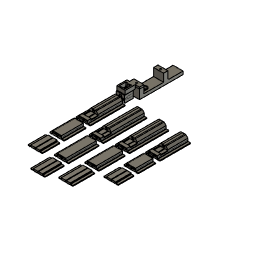
FlexiaGlove (Autodesk Fusion 360 design; units mm, degrees)
Autodesk Fusion 360 part; units mm, degrees
note: some values were not read from the file. Chosen so that the rebuilt part matches the saved one: which face or edge a step refers to. Set by a fixed rule: which sketch regions a step uses.
(part 1 of 2)
sketch "Sketch1" plane through (0, 0, 0) normal (0, 0, 1) x (1, 0, 0) in component "Flex Sensor Mount"
  line L0 (-4.7625, -1.75) -> (4.7625, -1.75)
  line L1 (4.7625, -1.75) -> (4.7625, 6.2)
  line L2 (-4.7625, 6.2) -> (-4.7625, -1.75)
  line L3 (-0.3, 0.4) -> (0.3, 0.4)
  line L4 (0.3, 0.4) -> (0.3, -0.4)
  line L5 (0.3, -0.4) -> (-0.3, -0.4)
  line L6 (-0.3, -0.4) -> (-0.3, 0.4)
  line L7 (-4.0625, 3.25) -> (4.0625, 3.25)
  line L8 (4.0625, 3.25) -> (4.0625, 0.75)
  line L9 (4.0625, 0.75) -> (-4.0625, 0.75)
  line L10 (-4.0625, 0.75) -> (-4.0625, 3.25)
  line L11 (-4.7625, 6.2) -> (4.7625, 6.2)
  dimension "d283" = 0.8
  dimension "d284" = 0.6
  dimension "d285" = 0.3
  dimension "d286" = 0.4
  dimension "d287" = 2.5
  dimension "d289" = 4.7625
  dimension "d291" = 1.75
  dimension "d293" = 0.35
  dimension "d294" = 8.125
  dimension "d296" = 9.525
  dimension "d297" = 4.0625
  dimension "d368" = 7.95
  constraint horizontal L0
  constraint vertical L1
  constraint vertical L2
  constraint horizontal L3
  constraint vertical L4
  constraint horizontal L5
  constraint vertical L6
  constraint horizontal L7
  constraint vertical L8
  constraint horizontal L9
  constraint vertical L10
  constraint horizontal L11
  measures "d283" distance of L3.start L5.end
  measures "d284" distance of L4.end L5.end
  measures "d285" distance of origin L6
  measures "d286" distance of origin L3
  measures "d287" distance of L7.end L8.end
  measures "d289" distance of origin L2
  measures "d291" distance of origin L0
  measures "d293" distance of L3 L9
  measures "d294" distance of L7.start L7.end
  measures "d296" distance of L0.start L0.end
  measures "d297" distance of origin L10
  measures "d368" distance of L0 L11
extrude "Extrude1" add sketch "Sketch1" along normal blind 12 from surface at 40.25 makes body 1 in component "Flex Sensor Mount"
sketch "Sketch3" plane through (0, 0, 52.25) normal (0, 0, 1) x (1, 0, 0) in component "Flex Sensor Mount"
  line L0 (0.3, -0.4) -> (-0.3, -0.4)
  line L1 (-0.3, -0.4) -> (-0.3, 0.4)
  line L2 (-0.3, 0.4) -> (0.3, 0.4)
  line L3 (0.3, 0.4) -> (0.3, -0.4)
  line L4 (4.0625, 0.75) -> (-4.0625, 0.75)
  line L5 (-4.0625, 0.75) -> (-4.0625, 3.25)
  line L6 (-4.0625, 3.25) -> (4.0625, 3.25)
  line L7 (4.0625, 3.25) -> (4.0625, 0.75)
  line L8 (-4.7625, 6.2) -> (-4.7625, -1.75)
  line L9 (-4.7625, -1.75) -> (4.7625, -1.75)
  line L10 (4.7625, -1.75) -> (4.7625, 6.2)
  line L11 (-4.0625, 2.5) -> (4.0625, 2.5)
  line L12 (4.0625, 2.5) -> (4.0625, 1.25)
  line L13 (4.0625, 1.25) -> (-4.0625, 1.25)
  line L14 (-4.0625, 1.25) -> (-4.0625, 2.5)
  line L15 (4.7625, 6.2) -> (-4.7625, 6.2)
  dimension "d305" = 1.25
  dimension "d312" = 0.75
  constraint horizontal L11
  constraint vertical L12
  constraint horizontal L13
  constraint vertical L14
  constraint coincident L7 L12.end
  constraint coincident L5 L11.start
  measures "d305" distance of L11.start L13.end
  measures "d312" distance of L6 L11
extrude "Extrude3" add sketch "Sketch3" against normal blind 4 contours L4 L5 L7 L13 | L5 L6 L7 L11 bodies 1 in component "Flex Sensor Mount"
sketch "Sketch2" plane through (0, 6.2, 0) normal (0, 1, 0) x (-1, 0, 0) in component "Flex Sensor Mount"
  line L0 (-4.7625, 40.25) -> (4.7625, 40.25)
  line L1 (4.7625, 40.25) -> (4.7625, 52.25)
  line L2 (4.7625, 52.25) -> (-4.7625, 52.25)
  line L3 (-4.7625, 52.25) -> (-4.7625, 40.25)
  line L4 (-4.0625, 40.25) -> (4.0625, 40.25)
  line L5 (4.0625, 40.25) -> (4.0625, 48.25)
  line L6 (-4.0625, 48.25) -> (-4.0625, 40.25)
  line L7 (4.0625, 52.25) -> (-4.0625, 52.25)
  line L8 (4.7625, 42.25) -> (-4.7625, 42.25)
  circle A0 centre (0, 46.9204) radius 6.6704
  line L9 (4.0625, 48.25) -> (-4.0625, 48.25)
  line L10 (-4.7625, 40.25) -> (4.7625, 40.25)
  line L11 (4.7625, 40.25) -> (4.7625, 52.25)
  line L12 (4.7625, 52.25) -> (-4.7625, 52.25)
  line L13 (-4.7625, 52.25) -> (-4.7625, 40.25)
  dimension "d302" = 2
  constraint coincident L5 L7.start
  constraint coincident L6 L7.end
  constraint perpendicular L6 L7
  constraint coincident L1 L8.start
  constraint coincident L3 L8.end
  constraint perpendicular L3 L8
  constraint coincident L8.start A0
  constraint tangent L0 A0
  constraint coincident L8.end A0
  measures "d302" distance of L0 L8
extrude "Extrude2" cut sketch "Sketch2" against normal up to surface (7.95 mm away) contours L0 L3 L6 A0 L10 L13 | L0 L4 L6 A0 L10 | L0 L4 L5 A0 L10 | L0 L1 L5 A0 L10 L11 bodies 1 in component "Flex Sensor Mount"
sketch "Sketch4" plane through (0, 6.2, 0) normal (0, 1, 0) x (-1, 0, 0) in component "Flex Sensor Mount"
  arc A0 (-4.7625, 42.25) -> (4.7625, 42.25) centre (0, 46.9204) ccw
  line L0 (4.7625, 42.25) -> (4.7625, 52.25)
  line L1 (4.7625, 52.25) -> (-4.7625, 52.25)
  line L2 (-4.7625, 52.25) -> (-4.7625, 42.25)
  circle A1 centre (0, 46.9204) radius 3.25
  line L3 (2.3452, 44.6704) -> (-2.3452, 44.6704)
  arc A2 (-4.7625, 42.25) -> (4.7625, 42.25) centre (0, 46.9204) ccw
  line L4 (4.7625, 42.25) -> (4.7625, 52.25)
  line L5 (4.7625, 52.25) -> (-4.7625, 52.25)
  line L6 (-4.7625, 52.25) -> (-4.7625, 42.25)
  dimension "d313" = 6.5
  dimension "d314" = 2.25
  constraint concentric A0 A1
  constraint coincident A1 L3.start
  constraint coincident A1 L3.end
  constraint horizontal L3
  measures "d313" diameter of A1
  measures "d314" distance of A0.centre L3
extrude "Extrude4" cut sketch "Sketch4" against normal blind 2.5 contours A1 L3 picked at (0.4352, 46.4124) bodies 1 in component "Flex Sensor Mount"
chamfer "Chamfer1" distance 0.1 angle 45 2 edges at (0, 6.2, 50.1704) (0, 6.2, 44.6704) on bodies 1 in component "Flex Sensor Mount"
sketch "Sketch1 (2)" plane through (0, 0, 0) normal (0, 0, 1) x (1, 0, 0) in component "Base"
  line L0 (-1.75, 1.75) -> (9.75, 1.75)
  line L1 (9.75, 1.75) -> (9.75, -1.75)
  line L2 (9.75, -1.75) -> (-1.75, -1.75)
  line L3 (-1.75, -1.75) -> (-1.75, 1.75)
  line L4 (-1.75, 1) -> (-0.25, 1)
  line L5 (-0.25, 1) -> (-0.25, -0.75)
  line L6 (-0.25, -0.75) -> (-1.75, -0.75)
  line L7 (-1.75, -0.75) -> (-1.75, 1)
  line L8 (9.75, 1) -> (8.25, 1)
  line L9 (8.25, 1) -> (8.25, -0.75)
  line L10 (8.25, -0.75) -> (9.75, -0.75)
  line L11 (9.75, -0.75) -> (9.75, 1)
  line L12 (-0.3, 0.4) -> (0.3, 0.4)
  line L13 (0.3, 0.4) -> (0.3, -0.4)
  line L14 (0.3, -0.4) -> (-0.3, -0.4)
  line L15 (-0.3, -0.4) -> (-0.3, 0.4)
  dimension "d1" = 11.5
  dimension "d4" = 1.75
  dimension "d77" = 1.75
  dimension "d79" = 1.5
  dimension "d80" = 1.75
  dimension "d81" = 1.5
  dimension "d83" = 1
  dimension "d84" = 1
  dimension "d86" = 3.5
  dimension "d87" = 1.75
  dimension "d131" = 0.6
  dimension "d132" = 0.8
  dimension "d133" = 0.3
  dimension "d134" = 0.4
  constraint horizontal L0
  constraint vertical L1
  constraint horizontal L2
  constraint vertical L3
  constraint horizontal L4
  constraint vertical L5
  constraint horizontal L6
  constraint vertical L7
  constraint coincident L3 L4.start
  constraint horizontal L8
  constraint vertical L9
  constraint horizontal L10
  constraint vertical L11
  constraint coincident L1 L8.start
  constraint horizontal L12
  constraint vertical L13
  constraint horizontal L14
  constraint vertical L15
  measures "d1" distance of L1.end L2.end
  measures "d4" distance of origin L3
  measures "d77" distance of L4.end L5.end
  measures "d79" distance of L4.start L4.end
  measures "d80" distance of L8.end L9.end
  measures "d81" distance of L8.start L8.end
  measures "d83" distance of L2 L10
  measures "d84" distance of L2 L6
  measures "d86" distance of L0 L2
  measures "d87" distance of origin L2
  measures "d131" distance of L12.start L12.end
  measures "d132" distance of L12.end L13.end
  measures "d133" distance of origin L15
  measures "d134" distance of origin L14
extrude "Extrude1'" add sketch "Sketch1 (2)" along normal blind 40 separate body contours L0 L1 L2 L3 L4 L5 L6 L8 L9 L10 L12 L13 L14 | L3 L4 L5 L6 L7 L12 L14 L15 | L1 L8 L9 L10 L11 makes body 2 in component "Base"
sketch "Sketch2 (2)" plane through (0, 1.75, 0) normal (0, 1, 0) x (-1, 0, 0) in component "Base"
  line L0 (-9.75, 0) -> (1.75, 0)
  line L1 (1.75, 0) -> (1.75, 40)
  line L2 (1.75, 40) -> (-9.75, 40)
  line L3 (-9.75, 40) -> (-9.75, 0)
  line L4 (-9.75, 40) -> (1.75, 40)
  line L5 (1.75, 40) -> (1.75, 35)
  line L6 (1.75, 35) -> (-9.75, 35)
  line L7 (-9.75, 35) -> (-9.75, 40)
  line L8 (-9.75, 12.4) -> (1.75, 12.4)
  line L9 (1.75, 12.4) -> (1.75, 7.4)
  line L10 (1.75, 7.4) -> (-9.75, 7.4)
  line L11 (-9.75, 7.4) -> (-9.75, 12.4)
  circle A0 centre (-4, 37.6385) radius 0.95
  circle A1 centre (-4, 10.0385) radius 0.95
  line L12 (-1.0736, 23.3752) -> (-1.0736, 24.3004)
  line L13 (-6.8236, 23.3752) -> (-6.8236, 24.241)
  arc A2 (-6.8236, 23.3752) -> (-1.0736, 23.3752) centre (-3.9486, 23.3752) ccw
  arc A3 (-1.0736, 24.3004) -> (-6.8236, 24.241) centre (-4, 29.25) ccw
  line L14 (-3.9486, 20.5002) -> (-4, 12.4)
  dimension "d8" = 11.5
  dimension "d9" = 11.5
  dimension "d10" = 5
  dimension "d11" = 5
  dimension "d12" = 27.6
  dimension "d13" = 22.6
  dimension "d15" = 5.75
  dimension "d16" = 5.75
  dimension "d17" = 1.9
  dimension "d18" = 1.9
  dimension "d47" = 5.75
  dimension "d48" = 11.5
  dimension "d49" = 5.75
  dimension "d50" = 5.875
  constraint horizontal L4
  constraint vertical L5
  constraint horizontal L6
  constraint vertical L7
  constraint coincident L2.end L3.start
  constraint horizontal L8
  constraint vertical L9
  constraint horizontal L10
  constraint vertical L11
  constraint coincident L3 L8.start
  constraint tangent L6 A3
  constraint vertical L12
  constraint vertical L13
  constraint tangent L12 A2
  constraint tangent L13 A2
  constraint midpoint A2 L14.start
  constraint midpoint L8 L14.end
  measures "d8" distance of L5.end L6.end
  measures "d9" distance of L9.end L10.end
  measures "d10" distance of L8.start L10.end
  measures "d11" distance of L2.end L6.end
  measures "d12" distance of A0.centre A1.centre
  measures "d13" distance of L6 L8
  measures "d15" horizontal distance of L2.end A0.centre
  measures "d16" distance of L11 A1.centre
  measures "d17" diameter of A0
  measures "d18" diameter of A1
  measures "d47" distance of L3 A3.centre
  measures "d48" diameter of A3
  measures "d49" diameter of A2
  measures "d50" distance of A3.centre A2.centre
extrude "Extrude1''" add sketch "Sketch2 (2)" along normal blind 9 contours L1 L3 L8 L9 L10 L11 | L1 L2 L3 L4 L5 L6 L7 bodies 2 in component "Base"
sketch "Sketch4 (2)" plane through (0, 1.75, 0) normal (0, 1, 0) x (-1, 0, 0) in component "Base"
  line L0 (1.75, 12.4) -> (1.75, 35)
  line L1 (1.75, 35) -> (-9.75, 35)
  line L2 (-9.75, 35) -> (-9.75, 12.4)
  line L3 (0.3, 24.6) -> (-9.75, 24.6)
  line L4 (0.3, 34.9) -> (-9.75, 34.9)
  line L5 (0.3, 34.9) -> (0.3, 24.6)
  line L6 (-9.75, 28.9) -> (-4, 28.9)
  circle A0 centre (-4, 28.9) radius 2.375
  circle A1 centre (-4, 28.9) radius 2.875
  line L7 (-8.3, 24.6) -> (-8.3, 34.9)
  line L8 (-9.75, 12.4) -> (1.75, 12.4)
  circle A2 centre (-4, 28.9) radius 4.3
  line L9 (-0.75, 24.6) -> (-0.75, 34.9)
  circle A3 centre (-4, 28.9) radius 3.25
  line L10 (-0.9996, 30.149) -> (0.3, 32.4)
  line L11 (-7.25, 28.9) -> (-7.25, 34.9)
  line L12 (-0.9996, 30.149) -> (-4, 28.9)
  dimension "d119" = 0.3
  dimension "d121" = 5.75
  dimension "d122" = 4.75
  dimension "d124" = 4.3
  dimension "d125" = 5.75
  dimension "d126" = 6
  dimension "d130" = 8.6
  dimension "d135" = 16.5
  dimension "d203" = 0.75
  dimension "d216" = 6.5
  dimension "d217" = 2.5
  dimension "d230" = 150
  dimension "d237" = 142.601
  constraint horizontal L4
  constraint horizontal L3
  constraint coincident L2 L3.end
  constraint coincident L2 L4.end
  constraint vertical L5
  constraint coincident L2 L6.start
  constraint perpendicular L2 L6
  constraint coincident L6.end A0.centre
  constraint coincident L3 L7.start
  constraint coincident L4 L7.end
  constraint perpendicular L4 L7
  constraint concentric A1 A2
  constraint tangent L5 A2
  constraint coincident L3 L9.start
  constraint coincident L4 L9.end
  constraint perpendicular L4 L9
  constraint concentric A2 A3
  constraint coincident A3 L10.start
  constraint coincident L5 L10.end
  constraint coincident A3 L11.start
  constraint coincident L6 L11.start
  constraint coincident L4 L11.end
  constraint tangent A3 L11
  measures "d119" distance of origin L5
  measures "d121" distance of L6.start L6.end
  measures "d122" diameter of A0
  measures "d124" distance of L3 L6
  measures "d125" diameter of A1
  measures "d126" distance of L4 L6.end
  measures "d130" distance of L5 L7
  measures "d135" distance of L6.end L8
  measures "d203" distance of origin L9
  measures "d216" diameter of A3
  measures "d217" distance of L4 L10.end
  measures "d230" angle of L5 L10
  measures "d237" angle of L10 L12
extrude "Extrude3'" cut sketch "Sketch4 (2)" against normal blind 2.85 contours L4 A2 L9 L11 | L6 A1 A3 L12 | A2 L9 A3 L10 L11 | L6 A1 A3 L12 | L4 L5 A2 L9 L10 | L6 A0 A1 L12 | L6 A0 A1 L12 | A2 L9 L10 | L6 A0 L12 | L6 A0 L12 picked at (-0.5421, 31.0649) bodies 2 in component "Base"
extrude "Extrude14" cut 1 faces at (8.15, 10.75, 37.5462) along direction (0, -1, 0) blind 2 on bodies 2 bodies 2 in component "Base"
chamfer "Chamfer1'" distance 1 angle 45 1 edges at (4, 1.75, 7.4) on bodies 2 in component "Base"
sketch "Sketch1 (3)" plane through (0, 8.75, 0) normal (0, 1, 0) x (-1, 0, 0) in component "Splay Sensor Mount"
  circle A0 centre (-4, 37.6385) radius 0.95
  line L0 (-9.75, 35) -> (1.75, 35)
  line L1 (1.75, 35) -> (1.75, 40)
  line L2 (1.75, 40) -> (-9.75, 40)
  line L3 (-9.75, 40) -> (-9.75, 35)
extrude "Extrude1'''" add sketch "Sketch1 (3)" along normal blind 2 separate body makes body 3 in component "Splay Sensor Mount"
sketch "Sketch2 (3)" plane through (0, 0, 40) normal (0, 0, 1) x (1, 0, 0) in component "Splay Sensor Mount"
  line L0 (-1.75, 8.75) -> (9.75, 8.75)
  line L1 (9.75, 8.75) -> (9.75, 10.75)
  line L2 (9.75, 10.75) -> (-1.75, 10.75)
  line L3 (-1.75, 10.75) -> (-1.75, 8.75)
  line L4 (4.7625, 10.75) -> (-4.7625, 10.75)
  line L5 (-4.7625, 10.75) -> (-4.7625, 6.25)
  line L6 (-4.7625, 6.25) -> (4.7625, 6.25)
  line L7 (4.7625, 6.25) -> (4.7625, 10.75)
  dimension "d327" = 9.525
  dimension "d328" = 4.5
  dimension "d329" = 4.7625
  constraint horizontal L4
  constraint vertical L5
  constraint horizontal L6
  constraint vertical L7
  constraint coincident L2 L4.start
  measures "d327" distance of L4.start L4.end
  measures "d328" distance of L4.start L6.end
  measures "d329" distance of origin L5
extrude "Extrude2'" add sketch "Sketch2 (3)" along normal blind 11.5 contours L0 L2 L3 L4 L7 | L0 L3 L4 L5 L6 L7 bodies 3 in component "Splay Sensor Mount"
sketch "Sketch3 (2)" plane through (0, 10.75, 0) normal (0, 1, 0) x (-1, 0, 0) in component "Splay Sensor Mount"
  circle A0 centre (-4, 37.6385) radius 0.95
  line L0 (-9.75, 40) -> (-9.75, 35)
  line L1 (-9.75, 35) -> (1.75, 35)
  line L2 (1.75, 35) -> (1.75, 40)
  line L3 (1.75, 40) -> (4.7625, 40)
  line L4 (4.7625, 40) -> (4.7625, 51.5)
  line L5 (4.7625, 51.5) -> (-4.7625, 51.5)
  line L6 (-4.7625, 51.5) -> (-4.7625, 40)
  line L7 (-4.7625, 40) -> (-9.75, 40)
  line L8 (3.25, 42.6704) -> (-3.25, 42.6704)
  line L9 (-3.25, 42.6704) -> (-3.25, 50.1704)
  line L10 (-3.25, 50.1704) -> (3.25, 50.1704)
  line L11 (3.25, 50.1704) -> (3.25, 42.6704)
  line L12 (3.25, 42.6704) -> (1, 42.6704)
  line L13 (1, 42.6704) -> (1, 43.4204)
  line L14 (1, 43.4204) -> (3.25, 43.4204)
  line L15 (3.25, 43.4204) -> (3.25, 42.6704)
  line L16 (-3.25, 42.6704) -> (-1, 42.6704)
  line L17 (-1, 42.6704) -> (-1, 43.4204)
  line L18 (-1, 43.4204) -> (-3.25, 43.4204)
  line L19 (-3.25, 43.4204) -> (-3.25, 42.6704)
  line L20 (1, 43.4204) -> (-1, 43.4204)
  arc A1 (2.3452, 44.6704) -> (-2.3452, 44.6704) centre (0, 46.9204) ccw
  dimension "d332" = 6.5
  dimension "d333" = 7.5
  dimension "d340" = 0.75
  dimension "d341" = 0.75
  dimension "d342" = 2
  dimension "d343" = 2.25
  dimension "d369" = 3.25
  dimension "d370" = 3.25
  constraint horizontal L8
  constraint vertical L9
  constraint horizontal L10
  constraint vertical L11
  constraint horizontal L12
  constraint vertical L13
  constraint horizontal L14
  constraint vertical L15
  constraint horizontal L16
  constraint vertical L17
  constraint horizontal L18
  constraint vertical L19
  measures "d332" distance of L9.end L10.end
  measures "d333" distance of L8.end L9.end
  measures "d340" distance of L16.end L17.end
  measures "d341" distance of L12.end L13.end
  measures "d342" distance of L13 L17
  measures "d343" distance of L13.end L14.end
  measures "d369" distance of L10 A1.centre
  measures "d370" distance of L11 A1.centre
extrude "Extrude3''" cut sketch "Sketch3 (2)" against normal up to surface (4.5 mm away) contours L8 L11 L12 L13 L14 L15 | L9 L11 L14 L18 L20 A1 | L8 L9 L16 L17 L18 L19 | L10 L11 A1 | L9 L10 A1 bodies 3 in component "Splay Sensor Mount"
sketch "Sketch1 (4)" plane through (0, 0, 0) normal (0, 1, 0) x (1, 0, 0) in component "Cam"
  circle A0 centre (4, -28.9) radius 2.375
  circle A1 centre (4, -28.9) radius 3.125
  line L0 (6.0041, -25.9523) -> (6.7835, -27.4795)
  line L1 (1.9959, -25.9523) -> (1.2165, -27.4795)
  line L2 (4, -28.9) -> (4, -26.975)
  line L3 (4, -28.9) -> (4, -32.525)
  line L4 (6.1835, -33.0681) -> (7.0326, -29.6543)
  line L5 (1.8165, -33.0681) -> (0.9674, -29.6543)
  arc A2 (6.0041, -25.9523) -> (1.9959, -25.9523) centre (4, -26.975) ccw
  arc A3 (1.8165, -33.0681) -> (6.1835, -33.0681) centre (4, -32.525) ccw
  arc A4 (7.25, -28.9) -> (0.9996, -30.149) centre (4, -28.9) ccw
  line L6 (0.9996, -30.149) -> (4, -28.9)
  line L7 (4, -28.9) -> (1.4251, -30.883)
  line L8 (-0.3, -32.4) -> (0.9996, -30.149)
  line L9 (0.0996, -31.7079) -> (0.0996, -39.0062)
  line L10 (0.9623, -32.6225) -> (1.5485, -34.7948)
  line L11 (1.5485, -34.7948) -> (4.0181, -34.7749)
  circle A5 centre (4, -28.9) radius 3.25
  line L12 (0.9623, -32.6225) -> (1.4661, -30.7289)
  dimension "d65" = 28.9
  dimension "d66" = 4
  dimension "d67" = 4.75
  dimension "d127" = 6.25
  dimension "d128" = 1.925
  dimension "d200" = 3.625
  dimension "d201" = 2.25
  dimension "d202" = 2.25
  dimension "d218" = 15
  dimension "d225" = 1.8
  dimension "d227" = 0.3996
  dimension "d232" = 1.8
  dimension "d234" = 2.25
  dimension "d235" = 150
  dimension "d238" = 142.5
  constraint concentric A0 A1
  constraint coincident A1 L0.end
  constraint coincident A1 L1.end
  constraint tangent A1 L1
  constraint tangent A1 L0
  constraint coincident A0.centre A1.centre
  constraint vertical L2
  constraint vertical L3
  constraint coincident A1 L4.end
  constraint coincident A1 L5.end
  constraint tangent A1 L5
  constraint tangent A1 L4
  constraint coincident L2.end A2.centre
  constraint coincident L3.end A3.centre
  constraint tangent L4 A3
  constraint tangent L5 A3
  constraint tangent L1 A2
  constraint tangent L0 A2
  constraint coincident A4.end L6.start
  constraint vertical L9
  constraint coincident L8 L9.start
  constraint coincident A3 L11.end
  constraint tangent A3 L11
  constraint concentric A1 A5
  constraint coincident A4.end A5
  constraint coincident A5 L7.end
  constraint coincident A1 L12.end
  constraint coincident L7.end L12
  measures "d65" vertical distance of origin A0.centre
  measures "d66" horizontal distance of origin A0.centre
  measures "d67" diameter of A0
  measures "d127" diameter of A1
  measures "d128" distance of A0.centre L2.end
  measures "d201" radius of A2
  measures "d202" radius of A3
  measures "d218" angle of L6 L7
  measures "d225" distance of A4.end L9.start
  measures "d227" distance of L8.start L9
  measures "d232" distance of L7.end L10.start
  measures "d234" distance of L10.start L10.end
  measures "d235" angle of L10 L12
  measures "d238" angle of L7 L12
extrude "Extrude1''''" add sketch "Sketch1 (4)" along normal blind 1.625 and the other way blind 1.125 from surface at 0.125 separate body contours A0 A1 L3 L6 | A0 A1 L6 L7 | A0 A1 L3 L7 | A1 L3 L7 A5 | A1 L3 L4 A5 | A1 L7 L12 | L4 L5 A3 A5 L12 | L5 A3 L10 L11 L12 makes body 4 in component "Cam"
sketch "Sketch5" plane through (0, 6.25, 0) normal (0, -1, 0) x (1, 0, 0) in component "Splay Sensor Mount"
  line L0 (-1, 42.6704) -> (-3.25, 42.6704)
  line L1 (-3.25, 42.6704) -> (-3.25, 50.1704)
  line L2 (-3.25, 50.1704) -> (3.25, 50.1704)
  line L3 (3.25, 50.1704) -> (3.25, 42.6704)
  line L4 (3.25, 42.6704) -> (1, 42.6704)
  line L5 (1, 42.6704) -> (1, 43.4204)
  line L6 (1, 43.4204) -> (-1, 43.4204)
  line L7 (-1, 43.4204) -> (-1, 42.6704)
  line L8 (-4.7625, 40) -> (4.7625, 40)
  line L9 (4.7625, 40) -> (4.7625, 51.5)
  line L10 (4.7625, 51.5) -> (-4.7625, 51.5)
  line L11 (-4.7625, 51.5) -> (-4.7625, 40)
  line L12 (-1, 43.4204) -> (-3.25, 43.4204)
  line L13 (-3.25, 43.4204) -> (-3.25, 42.6704)
  line L14 (-3.25, 42.6704) -> (-1, 42.6704)
  line L15 (-1, 42.6704) -> (-1, 43.4204)
  line L16 (1, 43.4204) -> (3.25, 43.4204)
  line L17 (3.25, 43.4204) -> (3.25, 42.6704)
  line L18 (3.25, 42.6704) -> (1, 42.6704)
  line L19 (1, 42.6704) -> (1, 43.4204)
  constraint horizontal L12
  constraint vertical L13
  constraint horizontal L14
  constraint vertical L15
  constraint coincident L0.end L1.start
  constraint coincident L6.end L7.start
  constraint horizontal L16
  constraint vertical L17
  constraint horizontal L18
  constraint vertical L19
  constraint coincident L3.end L4.start
  constraint coincident L5.end L6.start
extrude "Extrude5" add sketch "Sketch5" against normal blind 0.5 contours L0 L1 L7 L12 L13 L14 L15 | L3 L4 L5 L16 L17 L18 L19 bodies 3 in component "Splay Sensor Mount"
extrude "Extrude15" add 1 faces at (6.6, -0.1333, 0) along direction (0, 0, -1) blind 10 on bodies 2 bodies 2 in component "Base"
sketch "Sketch5 (2)" plane through (0, -1.75, 0) normal (0, -1, 0) x (1, 0, 0) in component "Flex Sensor Mount"
  arc A0 (-4.7625, 42.25) -> (4.7625, 42.25) centre (0, 46.9204) ccw
  line L0 (4.7625, 42.25) -> (4.7625, 52.25)
  line L1 (4.7625, 52.25) -> (-4.7625, 52.25)
  line L2 (-4.7625, 52.25) -> (-4.7625, 42.25)
  line L3 (-4.7625, 45.25) -> (4.7625, 45.25)
  line L4 (-1.5, 52.25) -> (1.5, 52.25)
  line L5 (1.5, 52.25) -> (1.5, 45.25)
  line L6 (1.5, 45.25) -> (-1.5, 45.25)
  line L7 (-1.5, 45.25) -> (-1.5, 52.25)
  dimension "d357" = 7
  dimension "d358" = 3
  dimension "d359" = 1.5
  constraint coincident L2 L3.start
  constraint coincident L0 L3.end
  constraint perpendicular L0 L3
  constraint horizontal L4
  constraint vertical L5
  constraint horizontal L6
  constraint vertical L7
  constraint coincident L3 L5.end
  constraint coincident L1 L4.start
  measures "d357" distance of L1 L6
  measures "d358" distance of L5 L7
  measures "d359" distance of origin L7
extrude "Extrude5'" cut sketch "Sketch5 (2)" against normal up to surface (2.15 mm away) contours L1 L3 L4 L5 L6 L7 bodies 1 in component "Flex Sensor Mount"
sketch "Sketch6" plane through (0, 0, 45.25) normal (0, 0, 1) x (1, 0, 0) in component "Flex Sensor Mount"
  line L0 (0.3, 0.4) -> (0.3, -0.4)
  line L1 (0.3, -0.4) -> (-0.3, -0.4)
  line L2 (-0.3, -0.4) -> (-0.3, 0.4)
  line L3 (-0.3, 0.4) -> (-1.5, 0.4)
  line L4 (-1.5, 0.4) -> (-1.5, -1.75)
  line L5 (-1.5, -1.75) -> (1.5, -1.75)
  line L6 (1.5, -1.75) -> (1.5, 0.4)
  line L7 (1.5, 0.4) -> (0.3, 0.4)
  line L8 (-1.5, -0.4) -> (1.5, -0.4)
  line L9 (1.5, -0.4) -> (1.5, 0.4)
  line L10 (1.5, 0.4) -> (-1.5, 0.4)
  line L11 (-1.5, 0.4) -> (-1.5, -0.4)
  constraint horizontal L8
  constraint vertical L9
  constraint horizontal L10
  constraint vertical L11
  constraint coincident L6.end L7.start
  constraint coincident L4 L8.start
extrude "Extrude6" cut sketch "Sketch6" along normal up to surface contours L0 L6 L7 L8 L9 L10 | L2 L3 L4 L8 L10 L11 end surface at (4.5389, 2.5667, 42.0324) on bodies 1 bodies 1 in component "Flex Sensor Mount"
fillet "Fillet2" radius 3 1 edges at (0, -0.4, 45.25) on bodies 1 in component "Flex Sensor Mount"
sketch "Sketch11" plane through (0, 0, 52.25) normal (0, 0, 1) x (1, 0, 0) in component "Flex Sensor Mount"
  line L0 (1.5, 0.4) -> (1.5, -1.75)
  line L1 (1.5, -1.75) -> (4.7625, -1.75)
  line L2 (4.7625, -1.75) -> (4.7625, 6.2)
  line L3 (4.7625, 6.2) -> (-4.7625, 6.2)
  line L4 (-4.7625, 6.2) -> (-4.7625, -1.75)
  line L5 (-4.7625, -1.75) -> (-1.5, -1.75)
  line L6 (-1.5, -1.75) -> (-1.5, 0.4)
  line L7 (-1.5, 0.4) -> (1.5, 0.4)
  line L8 (-4.0625, 1.25) -> (-4.0625, 2.5)
  line L9 (-4.0625, 2.5) -> (4.0625, 2.5)
  line L10 (4.0625, 2.5) -> (4.0625, 1.25)
  line L11 (4.0625, 1.25) -> (-4.0625, 1.25)
  line L12 (1.3125, 3.2) -> (1.3125, 4.7)
  line L13 (1.3125, 4.7) -> (-1.3125, 4.7)
  line L14 (-1.3125, 4.7) -> (-1.3125, 3.2)
  line L15 (-1.3125, 3.2) -> (1.3125, 3.2)
  dimension "d371" = 2.625
  dimension "d372" = 1.3125
  dimension "d373" = 1.5
  dimension "d377" = 0.7
  constraint vertical L12
  constraint horizontal L13
  constraint vertical L14
  measures "d371" distance of L12.end L13.end
  measures "d372" distance of origin L14
  measures "d373" distance of L12.start L12.end
  measures "d377" distance of L9 L15
extrude "Extrude7" cut sketch "Sketch11" against normal blind 2 contours L12 L13 L14 L15 bodies 1 in component "Flex Sensor Mount"
sketch "Sketch1 (5)" plane through (0, 0, 0) normal (0, 1, 0) x (1, 0, 0) in component "Finger Guides"
  line L0 (-8.2, -55) -> (8.2, -55)
  line L1 (8.2, -55) -> (8.2, -95)
  line L2 (8.2, -95) -> (-8.2, -95)
  line L3 (-8.2, -95) -> (-8.2, -55)
  line L4 (-8.2, -100) -> (8.2, -100)
  line L5 (8.2, -100) -> (8.2, -125)
  line L6 (8.2, -125) -> (-8.2, -125)
  line L7 (-8.2, -125) -> (-8.2, -100)
  line L8 (-8.2, -130) -> (8.2, -130)
  line L9 (8.2, -130) -> (8.2, -150)
  line L10 (8.2, -150) -> (-8.2, -150)
  line L11 (-8.2, -150) -> (-8.2, -130)
  line L12 (16.8, -110) -> (33.2, -110)
  line L13 (33.2, -105) -> (16.8, -105)
  line L14 (16.8, -105) -> (16.8, -55)
  line L15 (33.2, -145) -> (16.8, -145)
  line L16 (33.2, -172) -> (16.8, -172)
  line L17 (33.2, -110) -> (33.2, -145)
  line L18 (16.8, -172) -> (16.8, -150)
  line L19 (16.8, -55) -> (33.2, -55)
  line L20 (33.2, -150) -> (33.2, -172)
  line L21 (33.2, -55) -> (33.2, -105)
  line L22 (16.8, -150) -> (33.2, -150)
  line L23 (16.8, -145) -> (16.8, -110)
  line L24 (41.8, -165) -> (41.8, -140)
  line L25 (58.2, -135) -> (41.8, -135)
  line L26 (58.2, -105) -> (58.2, -135)
  line L27 (58.2, -165) -> (41.8, -165)
  line L28 (41.8, -105) -> (58.2, -105)
  line L29 (58.2, -55) -> (58.2, -100)
  line L30 (41.8, -140) -> (58.2, -140)
  line L31 (41.8, -55) -> (58.2, -55)
  line L32 (41.8, -135) -> (41.8, -105)
  line L33 (58.2, -140) -> (58.2, -165)
  line L34 (41.8, -100) -> (41.8, -55)
  line L35 (58.2, -100) -> (41.8, -100)
  line L36 (66.8, -138) -> (66.8, -120)
  line L37 (83.2, -115) -> (66.8, -115)
  line L38 (83.2, -95) -> (83.2, -115)
  line L39 (83.2, -138) -> (66.8, -138)
  line L40 (66.8, -95) -> (83.2, -95)
  line L41 (83.2, -55) -> (83.2, -90)
  line L42 (66.8, -120) -> (83.2, -120)
  line L43 (66.8, -55) -> (83.2, -55)
  line L44 (66.8, -115) -> (66.8, -95)
  line L45 (83.2, -120) -> (83.2, -138)
  line L46 (66.8, -90) -> (66.8, -55)
  line L47 (83.2, -90) -> (66.8, -90)
  dimension "d378" = 16.4
  dimension "d381" = 40
  dimension "d382" = 25
  dimension "d383" = 20
  dimension "d384" = 5
  dimension "d385" = 5
  dimension "d386" = 55
  dimension "d388" = 16.4
  dimension "d391" = 50
  dimension "d392" = 35
  dimension "d393" = 22
  dimension "d394" = 5
  dimension "d395" = 5
  dimension "d396" = 16.4
  dimension "d399" = 45
  dimension "d400" = 30
  dimension "d401" = 25
  dimension "d402" = 5
  dimension "d403" = 5
  dimension "d404" = 16.4
  dimension "d407" = 35
  dimension "d408" = 20
  dimension "d409" = 18
  dimension "d410" = 5
  dimension "d411" = 5
  constraint horizontal L0
  constraint vertical L1
  constraint horizontal L2
  constraint vertical L3
  constraint horizontal L4
  constraint vertical L5
  constraint horizontal L6
  constraint vertical L7
  constraint horizontal L8
  constraint vertical L9
  constraint horizontal L10
  constraint vertical L11
  constraint horizontal L19
  constraint vertical L21
  constraint horizontal L13
  constraint vertical L14
  constraint horizontal L12
  constraint vertical L17
  constraint horizontal L15
  constraint vertical L23
  constraint horizontal L22
  constraint vertical L20
  constraint horizontal L16
  constraint vertical L18
  constraint horizontal L31
  constraint vertical L29
  constraint horizontal L35
  constraint vertical L34
  constraint horizontal L28
  constraint vertical L26
  constraint horizontal L25
  constraint vertical L32
  constraint horizontal L30
  constraint vertical L33
  constraint horizontal L27
  constraint vertical L24
  constraint horizontal L43
  constraint vertical L41
  constraint horizontal L47
  constraint vertical L46
  constraint horizontal L40
  constraint vertical L38
  constraint horizontal L37
  constraint vertical L44
  constraint horizontal L42
  constraint vertical L45
  constraint horizontal L39
  constraint vertical L36
  constraint collinear L0 L19
  constraint collinear L19 L43
  constraint collinear L31 L43
  constraint collinear L3 L7
  constraint collinear L7 L11
  constraint collinear L5 L9
  constraint collinear L1 L5
  constraint collinear L18 L23
  constraint collinear L14 L23
  constraint collinear L17 L21
  constraint collinear L17 L20
  constraint collinear L24 L32
  constraint collinear L32 L34
  constraint collinear L26 L29
  constraint collinear L26 L33
  constraint collinear L36 L44
  constraint collinear L44 L46
  constraint collinear L38 L41
  constraint collinear L38 L45
  measures "d378" distance of L9.end L10.end
  measures "d381" distance of L0.start L2.end
  measures "d382" distance of L4.start L6.end
  measures "d383" distance of L8.start L10.end
  measures "d384" distance of L2 L4
  measures "d385" distance of L6 L8
  measures "d386" distance of origin L0
  measures "d388" distance of L16.end L16.start
  measures "d391" distance of L13.end L14.end
  measures "d392" distance of L15.end L12.start
  measures "d393" distance of L16.end L18.end
  measures "d394" distance of L12 L13
  measures "d395" distance of L15 L22
  measures "d396" distance of L27.start L24.start
  measures "d399" distance of L31.start L34.start
  measures "d400" distance of L25.end L28.start
  measures "d401" distance of L24.end L24.start
  measures "d402" distance of L28 L35
  measures "d403" distance of L25 L30
  measures "d404" distance of L39.start L36.start
  measures "d407" distance of L43.start L46.start
  measures "d408" distance of L37.end L40.start
  measures "d409" distance of L36.end L36.start
  measures "d410" distance of L40 L47
  measures "d411" distance of L37 L42
extrude "Extrude1'''''" add sketch "Sketch1 (5)" against normal blind 0.8 from surface at -0.4 separate body makes body 5 at (22.2667, -0.4, 121.6667) makes body 6 at (72.2667, -0.4, 126) makes body 7 at (22.2667, -0.4, 88.3333) makes body 8 at (47.2667, -0.4, 70) makes body 9 at (52.7333, -0.4, 125) makes body 10 at (2.7333, -0.4, 136.6667) makes body 11 at (27.7333, -0.4, 164.6667) makes body 12 at (77.7333, -0.4, 108.3333) makes body 13 at (-2.7333, -0.4, 68.3333) makes body 14 at (72.2667, -0.4, 66.6667) makes body 15 at (47.2667, -0.4, 148.3333) makes body 16 at (-2.7333, -0.4, 108.3333) in component "Finger Guides"
sketch "Sketch2 (4)" plane through (0, 0, 0) normal (0, 1, 0) x (1, 0, 0) in component "Finger Guides"
  line L0 (8.2, -95) -> (-8.2, -95)
  line L1 (8.2, -55) -> (8.2, -95)
  line L2 (-8.2, -55) -> (8.2, -55)
  line L3 (-8.2, -95) -> (-8.2, -55)
  line L4 (16.8, -55) -> (33.2, -55)
  line L5 (16.8, -105) -> (16.8, -55)
  line L6 (33.2, -105) -> (16.8, -105)
  line L7 (33.2, -55) -> (33.2, -105)
  line L8 (58.2, -55) -> (58.2, -100)
  line L9 (41.8, -55) -> (58.2, -55)
  line L10 (41.8, -100) -> (41.8, -55)
  line L11 (58.2, -100) -> (41.8, -100)
  line L12 (83.2, -55) -> (83.2, -90)
  line L13 (66.8, -55) -> (83.2, -55)
  line L14 (66.8, -90) -> (66.8, -55)
  line L15 (83.2, -90) -> (66.8, -90)
  line L16 (83.2, -115) -> (66.8, -115)
  line L17 (83.2, -95) -> (83.2, -115)
  line L18 (66.8, -95) -> (83.2, -95)
  line L19 (66.8, -115) -> (66.8, -95)
  line L20 (66.8, -120) -> (83.2, -120)
  line L21 (66.8, -138) -> (66.8, -120)
  line L22 (83.2, -138) -> (66.8, -138)
  line L23 (83.2, -120) -> (83.2, -138)
  line L24 (58.2, -135) -> (41.8, -135)
  line L25 (58.2, -105) -> (58.2, -135)
  line L26 (41.8, -105) -> (58.2, -105)
  line L27 (41.8, -135) -> (41.8, -105)
  line L28 (41.8, -140) -> (58.2, -140)
  line L29 (41.8, -165) -> (41.8, -140)
  line L30 (58.2, -165) -> (41.8, -165)
  line L31 (58.2, -140) -> (58.2, -165)
  line L32 (16.8, -172) -> (16.8, -150)
  line L33 (33.2, -172) -> (16.8, -172)
  line L34 (33.2, -150) -> (33.2, -172)
  line L35 (16.8, -150) -> (33.2, -150)
  line L36 (33.2, -145) -> (16.8, -145)
  line L37 (33.2, -110) -> (33.2, -145)
  line L38 (16.8, -110) -> (33.2, -110)
  line L39 (16.8, -145) -> (16.8, -110)
  line L40 (8.2, -125) -> (-8.2, -125)
  line L41 (8.2, -100) -> (8.2, -125)
  line L42 (-8.2, -100) -> (8.2, -100)
  line L43 (-8.2, -125) -> (-8.2, -100)
  line L44 (8.2, -150) -> (-8.2, -150)
  line L45 (8.2, -130) -> (8.2, -150)
  line L46 (-8.2, -130) -> (8.2, -130)
  line L47 (-8.2, -150) -> (-8.2, -130)
  line L48 (5.2, -55) -> (5.2, -95)
  line L49 (-5.2, -95) -> (-5.2, -55)
  line L50 (30.2, -55) -> (30.2, -105)
  line L51 (19.8, -105) -> (19.8, -55)
  line L52 (55.2, -55) -> (55.2, -100)
  line L53 (44.8, -100) -> (44.8, -55)
  line L54 (80.2, -55) -> (80.2, -90)
  line L55 (69.8, -90) -> (69.8, -55)
  line L56 (80.2, -95) -> (80.2, -115)
  line L57 (69.8, -115) -> (69.8, -95)
  line L58 (80.2, -120) -> (80.2, -138)
  line L59 (69.8, -138) -> (69.8, -120)
  line L60 (55.2, -105) -> (55.2, -135)
  line L61 (44.8, -135) -> (44.8, -105)
  line L62 (44.8, -140) -> (44.8, -165)
  line L63 (55.2, -165) -> (55.2, -140)
  line L64 (19.8, -150) -> (19.8, -172)
  line L65 (30.2, -172) -> (30.2, -150)
  line L66 (19.8, -145) -> (19.8, -110)
  line L67 (30.2, -110) -> (30.2, -145)
  line L68 (-5.2, -100) -> (-5.2, -125)
  line L69 (5.2, -125) -> (5.2, -100)
  line L70 (5.2, -130) -> (5.2, -150)
  line L71 (-5.2, -150) -> (-5.2, -130)
  dimension "d414" = 10.4
  dimension "d415" = 10.4
  dimension "d416" = 10.4
  dimension "d417" = 10.4
  dimension "d426" = 3
  dimension "d427" = 3
  dimension "d428" = 3
  dimension "d429" = 3
  constraint vertical L48
  constraint vertical L49
  constraint coincident L0 L48.end
  constraint coincident L2 L49.end
  constraint vertical L50
  constraint vertical L51
  constraint coincident L6 L50.end
  constraint coincident L4 L51.end
  constraint vertical L52
  constraint vertical L53
  constraint coincident L11 L52.end
  constraint coincident L9 L53.end
  constraint vertical L54
  constraint vertical L55
  constraint coincident L15 L54.end
  constraint coincident L13 L55.end
  constraint vertical L56
  constraint vertical L57
  constraint coincident L16 L56.end
  constraint coincident L18 L57.end
  constraint vertical L58
  constraint vertical L59
  constraint coincident L22 L58.end
  constraint coincident L20 L59.end
  constraint vertical L60
  constraint vertical L61
  constraint coincident L24 L60.end
  constraint coincident L26 L61.end
  constraint vertical L62
  constraint vertical L63
  constraint coincident L30 L62.end
  constraint coincident L28 L63.end
  constraint vertical L64
  constraint vertical L65
  constraint coincident L33 L64.end
  constraint coincident L35 L65.end
  constraint vertical L66
  constraint vertical L67
  constraint coincident L38 L66.end
  constraint coincident L36 L67.end
  constraint vertical L68
  constraint vertical L69
  constraint coincident L40 L68.end
  constraint coincident L42 L69.end
  constraint vertical L70
  constraint vertical L71
  constraint coincident L44 L70.end
  constraint coincident L46 L71.end
  constraint coincident L44 L71.start
  constraint coincident L46 L70.start
  constraint coincident L40 L69.start
  constraint coincident L42 L68.start
  constraint coincident L0 L49.start
  constraint coincident L2 L48.start
  constraint coincident L4 L50.start
  constraint coincident L6 L51.start
  constraint coincident L38 L67.start
  constraint coincident L36 L66.start
  constraint coincident L35 L64.start
  constraint coincident L33 L65.start
  constraint coincident L28 L62.start
  constraint coincident L30 L63.start
  constraint coincident L24 L61.start
  constraint coincident L26 L60.start
  constraint coincident L11 L53.start
  constraint coincident L9 L52.start
  constraint coincident L13 L54.start
  constraint coincident L15 L55.start
  constraint coincident L16 L57.start
  constraint coincident L20 L58.start
  constraint coincident L22 L59.start
  constraint collinear L68 L71
  constraint collinear L49 L68
  constraint collinear L51 L66
  constraint collinear L64 L66
  constraint collinear L61 L62
  constraint collinear L53 L61
  constraint collinear L52 L60
  constraint collinear L60 L63
  constraint collinear L57 L59
  constraint collinear L55 L57
  constraint collinear L54 L56
  constraint collinear L56 L58
  constraint collinear L50 L67
  constraint collinear L65 L67
  constraint collinear L69 L70
  constraint collinear L48 L69
  measures "d414" distance of L70 L71
  measures "d415" distance of L64 L65
  measures "d416" distance of L62 L63
  measures "d417" distance of L58 L59
  measures "d426" distance of L44.end L71.start
  measures "d427" distance of L32.start L64.end
  measures "d428" distance of L62.end L29.start
  measures "d429" distance of L59.start L21.start
extrude "Extrude2''" add sketch "Sketch2 (4)" along normal blind 3.1 from surface at -0.4 contours L0 L2 L48 L49 | L4 L6 L50 L51 | L9 L11 L52 L53 | L13 L15 L54 L55 | L16 L18 L56 L57 | L20 L22 L58 L59 | L24 L26 L60 L61 | L28 L30 L62 L63 | L33 L35 L64 L65 | L36 L38 L66 L67 | L40 L42 L68 L69 | L44 L46 L70 L71 bodies 5 6 7 8 9 10 11 12 13 14 15 16 in component "Finger Guides"
sketch "Sketch3 (3)" plane through (0, 0, 172) normal (0, 0, 1) x (1, 0, 0) in component "Finger Guides"
  line L0 (30.2, -0.4) -> (30.2, 2.7)
  line L1 (30.2, 2.7) -> (19.8, 2.7)
  line L2 (19.8, 2.7) -> (19.8, -0.4)
  line L3 (-0.3, 0.4) -> (0.3, 0.4)
  line L4 (0.3, 0.4) -> (0.3, -0.4)
  line L5 (0.3, -0.4) -> (-0.3, -0.4)
  line L6 (-0.3, -0.4) -> (-0.3, 0.4)
  line L7 (24.7, 0.4) -> (25.3, 0.4)
  line L8 (25.3, 0.4) -> (25.3, -0.4)
  line L9 (25.3, -0.4) -> (24.7, -0.4)
  line L10 (24.7, -0.4) -> (24.7, 0.4)
  line L11 (49.7, 0.4) -> (50.3, 0.4)
  line L12 (50.3, 0.4) -> (50.3, -0.4)
  line L13 (50.3, -0.4) -> (49.7, -0.4)
  line L14 (49.7, -0.4) -> (49.7, 0.4)
  line L15 (74.7, 0.4) -> (75.3, 0.4)
  line L16 (75.3, 0.4) -> (75.3, -0.4)
  line L17 (75.3, -0.4) -> (74.7, -0.4)
  line L18 (74.7, -0.4) -> (74.7, 0.4)
  line L19 (-4.5, 2) -> (4.5, 2)
  line L20 (4.5, 2) -> (4.5, 0.7)
  line L21 (4.5, 0.7) -> (-4.5, 0.7)
  line L22 (-4.5, 0.7) -> (-4.5, 2)
  line L23 (5.2, -0.4) -> (5.2, 2.7)
  line L24 (5.2, 2.7) -> (-5.2, 2.7)
  line L25 (-5.2, 2.7) -> (-5.2, -0.4)
  line L26 (8.2, -0.4) -> (5.2, -0.4)
  line L27 (-8.2, -0.4) -> (-8.2, -1.2)
  line L28 (-8.2, -1.2) -> (8.2, -1.2)
  line L29 (8.2, -1.2) -> (8.2, -0.4)
  line L30 (33.2, -0.4) -> (30.2, -0.4)
  line L31 (16.8, -0.4) -> (16.8, -1.2)
  line L32 (16.8, -1.2) -> (33.2, -1.2)
  line L33 (33.2, -1.2) -> (33.2, -0.4)
  line L34 (55.2, -0.4) -> (55.2, 2.7)
  line L35 (55.2, 2.7) -> (44.8, 2.7)
  line L36 (44.8, 2.7) -> (44.8, -0.4)
  line L37 (58.2, -0.4) -> (55.2, -0.4)
  line L38 (41.8, -0.4) -> (41.8, -1.2)
  line L39 (41.8, -1.2) -> (58.2, -1.2)
  line L40 (58.2, -1.2) -> (58.2, -0.4)
  line L41 (80.2, -0.4) -> (80.2, 2.7)
  line L42 (80.2, 2.7) -> (69.8, 2.7)
  line L43 (69.8, 2.7) -> (69.8, -0.4)
  line L44 (83.2, -0.4) -> (80.2, -0.4)
  line L45 (66.8, -0.4) -> (66.8, -1.2)
  line L46 (66.8, -1.2) -> (83.2, -1.2)
  line L47 (83.2, -1.2) -> (83.2, -0.4)
  line L48 (20.5, 2) -> (29.5, 2)
  line L49 (29.5, 2) -> (29.5, 0.7)
  line L50 (29.5, 0.7) -> (20.5, 0.7)
  line L51 (20.5, 0.7) -> (20.5, 2)
  line L52 (45.5, 2) -> (54.5, 2)
  line L53 (54.5, 2) -> (54.5, 0.7)
  line L54 (54.5, 0.7) -> (45.5, 0.7)
  line L55 (45.5, 0.7) -> (45.5, 2)
  line L56 (70.5, 2) -> (79.5, 2)
  line L57 (79.5, 2) -> (79.5, 0.7)
  line L58 (79.5, 0.7) -> (70.5, 0.7)
  line L59 (70.5, 0.7) -> (70.5, 2)
  line L60 (-5.65, -1.2) -> (-5.2, -0.75)
  line L61 (-5.2, -0.75) -> (-4.75, -1.2)
  line L62 (4.75, -1.2) -> (5.2, -0.75)
  line L63 (5.2, -0.75) -> (5.65, -1.2)
  line L64 (19.35, -1.2) -> (19.8, -0.75)
  line L65 (19.8, -0.75) -> (20.25, -1.2)
  line L66 (29.75, -1.2) -> (30.2, -0.75)
  line L67 (30.2, -0.75) -> (30.65, -1.2)
  line L68 (44.35, -1.2) -> (44.8, -0.75)
  line L69 (44.8, -0.75) -> (45.25, -1.2)
  line L70 (54.75, -1.2) -> (55.2, -0.75)
  line L71 (55.2, -0.75) -> (55.65, -1.2)
  line L72 (69.35, -1.2) -> (69.8, -0.75)
  line L73 (69.8, -0.75) -> (70.25, -1.2)
  line L74 (79.75, -1.2) -> (80.2, -0.75)
  line L75 (80.2, -0.75) -> (80.65, -1.2)
  line L76 (33.2, -0.4) -> (30.2, -0.4)
  line L77 (19.8, -0.4) -> (16.8, -0.4)
  line L78 (16.8, -0.4) -> (16.8, -1.2)
  line L79 (16.8, -1.2) -> (33.2, -1.2)
  line L80 (33.2, -1.2) -> (33.2, -0.4)
  line L81 (8.2, -0.4) -> (5.2, -0.4)
  line L82 (-5.2, -0.4) -> (-8.2, -0.4)
  line L83 (-8.2, -0.4) -> (-8.2, -1.2)
  line L84 (-8.2, -1.2) -> (8.2, -1.2)
  line L85 (8.2, -1.2) -> (8.2, -0.4)
  line L86 (5.2, -0.4) -> (5.2, 2.7)
  line L87 (5.2, 2.7) -> (-5.2, 2.7)
  line L88 (-5.2, 2.7) -> (-5.2, -0.4)
  line L89 (-5.2, -0.4) -> (-8.2, -0.4)
  line L90 (30.2, -0.4) -> (30.2, 2.7)
  line L91 (30.2, 2.7) -> (19.8, 2.7)
  line L92 (19.8, 2.7) -> (19.8, -0.4)
  line L93 (19.8, -0.4) -> (16.8, -0.4)
  line L94 (58.2, -0.4) -> (55.2, -0.4)
  line L95 (44.8, -0.4) -> (41.8, -0.4)
  line L96 (41.8, -0.4) -> (41.8, -1.2)
  line L97 (41.8, -1.2) -> (58.2, -1.2)
  line L98 (58.2, -1.2) -> (58.2, -0.4)
  line L99 (55.2, -0.4) -> (55.2, 2.7)
  line L100 (55.2, 2.7) -> (44.8, 2.7)
  line L101 (44.8, 2.7) -> (44.8, -0.4)
  line L102 (44.8, -0.4) -> (41.8, -0.4)
  line L103 (83.2, -0.4) -> (80.2, -0.4)
  line L104 (69.8, -0.4) -> (66.8, -0.4)
  line L105 (66.8, -0.4) -> (66.8, -1.2)
  line L106 (66.8, -1.2) -> (83.2, -1.2)
  line L107 (83.2, -1.2) -> (83.2, -0.4)
  line L108 (80.2, -0.4) -> (80.2, 2.7)
  line L109 (80.2, 2.7) -> (69.8, 2.7)
  line L110 (69.8, 2.7) -> (69.8, -0.4)
  line L111 (69.8, -0.4) -> (66.8, -0.4)
  dimension "d431" = 0.8
  dimension "d432" = 0.6
  dimension "d433" = 0.3
  dimension "d434" = 0.4
  dimension "d435" = 0.7
  dimension "d436" = 0.7
  dimension "d437" = 0.7
  dimension "d438" = 4.9
  dimension "d439" = 0.8
  dimension "d440" = 0.8
  dimension "d441" = 4.9
  dimension "d442" = 0.8
  dimension "d443" = 4.9
  dimension "d444" = 4.9
  dimension "d445" = 0.8
  dimension "d446" = 0.6
  dimension "d447" = 0.8
  dimension "d448" = 0.8
  dimension "d449" = 0.6
  dimension "d450" = 0.8
  dimension "d451" = 0.6
  dimension "d452" = 0.7
  dimension "d453" = 0.7
  dimension "d454" = 0.7
  dimension "d455" = 0.7
  dimension "d456" = 0.7
  dimension "d457" = 0.7
  dimension "d458" = 0.7
  dimension "d459" = 0.7
  dimension "d460" = 0.7
  dimension "d461" = 0.45
  dimension "d462" = 0.45
  dimension "d463" = 0.45
  dimension "d464" = 0.45
  dimension "d465" = 0.45
  dimension "d466" = 0.45
  dimension "d467" = 0.45
  dimension "d468" = 0.45
  dimension "d476" = 45
  dimension "d484" = 1.3
  dimension "d485" = 1.3
  dimension "d486" = 1.3
  dimension "d487" = 1.3
  constraint horizontal L3
  constraint vertical L4
  constraint horizontal L5
  constraint vertical L6
  constraint horizontal L7
  constraint vertical L8
  constraint horizontal L9
  constraint vertical L10
  constraint horizontal L11
  constraint vertical L12
  constraint horizontal L13
  constraint vertical L14
  constraint horizontal L15
  constraint vertical L16
  constraint horizontal L17
  constraint vertical L18
  constraint horizontal L19
  constraint vertical L20
  constraint horizontal L21
  constraint vertical L22
  constraint horizontal L48
  constraint vertical L49
  constraint horizontal L50
  constraint vertical L51
  constraint horizontal L52
  constraint vertical L53
  constraint horizontal L54
  constraint vertical L55
  constraint horizontal L56
  constraint vertical L57
  constraint horizontal L58
  constraint vertical L59
  constraint coincident L28 L60.start
  constraint coincident L28 L61.end
  constraint coincident L28 L62.start
  constraint coincident L28 L63.end
  constraint coincident L32 L64.start
  constraint perpendicular L63 L64
  constraint coincident L32 L65.end
  constraint coincident L32 L66.start
  constraint coincident L32 L67.end
  constraint perpendicular L66 L67
  constraint coincident L39 L68.start
  constraint perpendicular L67 L68
  constraint coincident L39 L69.end
  constraint perpendicular L68 L69
  constraint perpendicular L69 L70
  constraint coincident L39 L71.end
  constraint perpendicular L70 L71
  constraint perpendicular L60 L61
  constraint coincident L46 L72.start
  constraint coincident L46 L73.end
  constraint coincident L46 L74.start
  constraint coincident L46 L75.end
  constraint perpendicular L74 L75
  constraint perpendicular L72 L73
  constraint coincident L39 L70.start
  constraint perpendicular L64 L65
  measures "d431" distance of L3.end L4.end
  measures "d432" distance of L3.start L3.end
  measures "d433" distance of origin L6
  measures "d434" distance of origin L3
  measures "d435" distance of L22 L25
  measures "d436" distance of L19 L24
  measures "d437" distance of L20 L23
  measures "d438" distance of L4 L23
  measures "d439" distance of L5.end L28
  measures "d440" distance of L9 L32
  measures "d441" distance of L0 L8
  measures "d442" distance of L13 L39
  measures "d443" distance of L12 L34
  measures "d444" distance of L16 L41
  measures "d445" distance of L17 L46
  measures "d446" distance of L15.start L15.end
  measures "d447" distance of L15.end L16.end
  measures "d448" distance of L11.end L12.end
  measures "d449" distance of L11.start L11.end
  measures "d450" distance of L7.end L8.end
  measures "d451" distance of L7.start L7.end
  measures "d452" distance of L1 L48
  measures "d453" distance of L2 L51
  measures "d454" distance of L0 L49
  measures "d455" distance of L42 L56
  measures "d456" distance of L43 L59
  measures "d457" distance of L41 L57
  measures "d458" distance of L34 L53
  measures "d459" distance of L35 L52
  measures "d460" distance of L36 L55
  measures "d461" distance of L39 L70.end
  measures "d462" distance of L39 L68.end
  measures "d463" distance of L32 L66.end
  measures "d464" distance of L32 L64.end
  measures "d465" distance of L28 L62.end
  measures "d466" distance of L28 L60.end
  measures "d467" distance of L46 L74.end
  measures "d468" distance of L46 L72.end
  measures "d476" angle of L39 L71
  measures "d484" distance of L19.end L20.end
  measures "d485" distance of L48.end L49.end
  measures "d486" distance of L52.end L53.end
  measures "d487" distance of L56.end L57.end
extrude "Extrude3'''" cut sketch "Sketch3 (3)" against normal up to surface (117 mm away) contours L32 L66 L67 L79 | L32 L64 L65 L79 | L3 L4 L5 L6 | L7 L8 L9 L10 | L11 L12 L13 L14 | L15 L16 L17 L18 | L19 L20 L21 L22 | L28 L62 L63 L84 | L28 L60 L61 L84 | L39 L70 L71 L97 | L39 L68 L69 L97 | L46 L74 L75 L106 | L46 L72 L73 L106 | L48 L49 L50 L51 | L52 L53 L54 L55 | L56 L57 L58 L59 bodies 5 6 7 8 9 10 11 12 13 14 15 16 in component "Finger Guides"